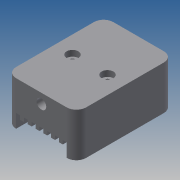
# Autodesk Inventor part: wire block
Saved by Autodesk Inventor 2013 (Build 170138000, 138)
## iProperties
Created: 2017-04-12
Part Number: wire block
Material: Generic
Document SubType Name: Modeling
Designer: employee
Density: 1 g/cm^3
Author: employee
Autodesk Inventor part; units mm, degrees
ref_plane "YZ Plane" through (0, 0, 0) normal (1, 0, 0) x (0, 1, 0)
ref_plane "XZ Plane" through (0, 0, 0) normal (0, 1, 0) x (-1, 0, 0)
ref_plane "XY Plane" through (0, 0, 0) normal (0, 0, 1) x (1, 0, 0)
sketch "Sketch1" plane through (0, 0, 0) normal (0, 0, 1) x (1, 0, 0)
  line L0 (-13, 20) -> (13, 20)
  line L1 (13, 20) -> (13, -20)
  line L2 (13, -20) -> (-13, -20)
  line L3 (-13, -20) -> (-13, 20)
  line L4 (18, 25) -> (-18, 25)
  line L5 (-18, 25) -> (-18, -25)
  line L6 (-18, -25) -> (18, -25)
  line L7 (18, -25) -> (18, 25)
  point P0 (0, 0)
  point P1 (-13, 0)
  point P2 (0, 20)
  dimension "d0" = 26
  dimension "d1" = 40
  dimension "d2" = 5
  constraints: 16 end point, 4 parallel, 2 midpoint, 2 perpendicular, 1 horizontal, 1 horizontal alignment, 1 vertical alignment, 3 other
  measures "d0" distance of L0.start L0.end
  measures "d1" distance of L2.end L0.start
  measures "d2" distance between parallel lines of L5 L3
extrude "Extrusion1" add sketch "Sketch1" along normal blind 12.5
sketch "Sketch3" plane through (0, 0, 12.5) normal (0, 0, 1) x (1, 0, 0)
  line L0 (-2.5, -25) -> (-2.5, -20) projected
  line L1 (13, -20) -> (-13, -20) projected
  line L2 (-13, -20) -> (-13, 20) projected
  line L3 (-13, 20) -> (13, 20) projected
  line L4 (-2.5, 20) -> (-2.5, 25) projected
  line L5 (18, 25) -> (-18, 25) projected
  line L6 (-18, 25) -> (-18, -25) projected
  line L7 (-18, -25) -> (18, -25) projected
  line L8 (-18, -25) -> (18, -25) projected
  line L9 (18, -25) -> (18, 25) projected
  line L10 (18, 25) -> (-18, 25) projected
  line L11 (-13, 20) -> (13, 20) projected
  line L12 (13, 20) -> (13, -20) projected
  line L13 (13, -20) -> (-13, -20) projected
  line L14 (-13, -20) -> (-13, 20) projected
  line L15 (-18, 25) -> (-18, -25) projected
  point P0 (0, 0)
extrude "Extrusion3" add sketch "Sketch3" along normal blind 5
sketch "Sketch4" plane through (0, 0, 0) normal (0, 0, -1) x (-1, 0, 0)
  line L0 (-13, 20) -> (13, 20) projected
  line L1 (-18, 25) -> (18, 25) projected
  line L2 (-10.5, 25) -> (10.5, 25)
  line L3 (10.5, 25) -> (10.5, 20)
  line L4 (10.5, 20) -> (-10.5, 20)
  line L5 (-10.5, 20) -> (-10.5, 25)
  point P0 (0, 0)
  point P1 (0, 25)
  point P2 (0, 25)
  dimension "d11" = 21
  constraints: 8 end point, 2 midpoint, 2 parallel, 2 point on line, 1 coincident, 1 horizontal, 1 perpendicular
  measures "d11" distance between parallel lines of L3 L5
extrude "Extrusion4" cut sketch "Sketch4" against normal blind 1
sketch "Sketch5" plane through (-18, -25, 0) normal (0, -1, 0) x (1, 0, 0)
  line L0 (0, 0) -> (36, 0) projected
  line L1 (17, 0) -> (19, 0)
  line L2 (19, 0) -> (19, 2)
  line L3 (19, 2) -> (17, 2)
  line L4 (17, 2) -> (17, 0)
  point P0 (18, 0)
  point P1 (18, 0)
  dimension "d15" = 2
  constraints: 8 end point, 2 midpoint, 2 parallel, 2 perpendicular, 1 horizontal, 1 point on line
  measures "d15" distance of L1.end L2.end
extrude "Extrusion5" cut sketch "Sketch5" against normal up to surface (45 mm away)
pattern_linear "Rectangular Pattern1" count 7 spacing 4 along (1, 0, 0) of "Extrusion5" first direction both ways yes
sketch "Sketch6" plane through (13, -25, 0) normal (0, -1, 0) x (1, 0, 0)
  circle A0 centre (-13, 12.5) radius 2.5
  point P0 (-13, 0)
  dimension "d22" = 12.5
  dimension "d23" = 5
  constraints: 1 centre point, 1 vertical alignment
  measures "d22" distance of point (-13, 0) A0.centre
  measures "d23" diameter of A0
extrude "Extrusion6" cut sketch "Sketch6" against normal through all
sketch "Sketch7" plane through (0, 0, 0) normal (0, 0, -1) x (-1, 0, 0)
  line L0 (-13, -25) -> (-13, 20) projected
  line L1 (-13, 20) -> (-10.5, 20) projected
  line L2 (-10.5, 20) -> (-10.5, 25) projected
  line L3 (-18, 25) -> (-10.5, 25) projected
  line L4 (-18, -25) -> (-18, 25) projected
  line L5 (-13, -25) -> (-18, -25) projected
  line L6 (-18, 25) -> (-13, 25)
  line L7 (-13, 25) -> (-13, -25)
  line L8 (-13, -25) -> (-18, -25)
  line L9 (-18, -25) -> (-18, 25)
  line L10 (13, -25) -> (18, -25)
  line L11 (18, -25) -> (18, 25)
  line L12 (18, 25) -> (13, 25)
  line L13 (13, 25) -> (13, -25)
  line L14 (-18, 25) -> (-10.5, 25) projected
  point P0 (0, 0)
  constraints: 16 end point, 4 parallel, 2 horizontal, 2 perpendicular, 2 point on line
extrude "Extrusion7" add sketch "Sketch7" along normal blind 5 contours L5 L4 L3 L7 L0 | L13 L12 L11 L10
fillet "Fillet3" radius 5 4 edges at (18, 25, 6.25) (18, -25, 6.25) (-18, -25, 6.25) (-18, 25, 6.25)
sketch "Sketch8" plane through (0, 0, 17.5) normal (0, 0, 1) x (1, 0, 0)
  circle A0 centre (-9, 0) radius 3
  point P0 (0, 0)
  dimension "d31" = 6
  dimension "d34" = 9
  constraints: 1 centre point, 1 horizontal alignment
  measures "d31" diameter of A0
  measures "d34" distance of point (0, 0) A0.centre
extrude "Extrusion8" cut sketch "Sketch8" against normal blind 3
sketch "Sketch9" plane through (-9, 0, 14.5) normal (0, 0, 1) x (1, 0, 0)
  circle A0 centre (0, 0) radius 3 projected
  circle A1 centre (0, 0) radius 1.75
  point P0 (9, 0)
  dimension "d37" = 3.5
  constraints: 1 centre point, 1 coincident
  measures "d37" diameter of A1
extrude "Extrusion9" cut sketch "Sketch9" against normal through all contours A1
mirror "Mirror1" about plane through (0, 0, 0) normal (1, 0, 0) of "Extrusion8", "Extrusion9"
body "Solid1"
